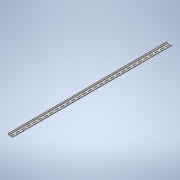
# Autodesk Inventor part: TrilhoDIN_Furado_1m
Saved by Autodesk Inventor 2021 (Build 250183000, 183)
## iProperties
Created: 2022-06-08
Part Number: TrilhoDIN_Furado_1m
Material: Generic
Document SubType Name: Sheet Metal
Designer: danie
Density: 1 g/cm^3
Sheet Metal Rule: Default_mm
Appearance: Default
Author: danie
Autodesk Inventor part; units mm, degrees
(part 1 of 2)
ref_plane "YZ Plane" through (0, 0, 0) normal (1, 0, 0) x (0, 1, 0)
ref_plane "XZ Plane" through (0, 0, 0) normal (0, 1, 0) x (-1, 0, 0)
ref_plane "XY Plane" through (0, 0, 0) normal (0, 0, 1) x (1, 0, 0)
sketch "Sketch1" plane through (0, 0, 0) normal (0, 1, 0) x (-1, 0, 0)
  line L0 (-13.5, 500) -> (13.5, 500)
  line L1 (13.5, 500) -> (13.5, -500)
  line L2 (13.5, -500) -> (-13.5, -500)
  line L3 (-13.5, -500) -> (-13.5, 500)
  line L4 (-13.5, 500) -> (13.5, -500) construction
  line L5 (13.5, 500) -> (-13.5, -500) construction
  point P0 (0, 0)
  dimension "d0" = 27
  dimension "d1" = 1000
  measures "d0" distance of L1.end L2.end
  measures "d1" distance of L0.end L1.end
extrude "Plate1" add sketch "Sketch1" along normal blind 1.5
sketch "Sketch2" plane through (12, 0, -500) normal (1, 0, 0) x (0, 1, 0)
  line L0 (0, 1000) -> (0, 0)
  line L1 (0, 0) -> (7.3, 0)
  line L2 (7.3, 0) -> (7.3, 1000)
  line L3 (7.3, 1000) -> (0, 1000)
  constraints: 6 end point, 1 horizontal, 1 perpendicular, 1 vertical
edge flange "Flange1" height 7.3 angle 90 thickness 1.5 bend radius 1.5 thickness toward (1, 0, 0) relief tear relief width 1.5 relief depth 0.75 corner gap 1.5 corner form 0 edges at (13.5, 1.5, 0) (-13.5, 1.5, 0) wall of the first edge with corners at (12, 0, 500) (12, 0, -500) (12, 7.3, -500) (12, 7.3, 500)
bend "Bend1"
corner "Corner1"
sketch "Sketch3" plane through (12, 5.8, 500) normal (0, 1, 0) x (-1, 0, 0)
  line L0 (0, -1000) -> (0, 0)
  line L1 (0, 0) -> (-5.5, 0)
  line L2 (-5.5, 0) -> (-5.5, -1000)
  line L3 (-5.5, -1000) -> (0, -1000)
  constraints: 6 end point, 1 horizontal, 1 perpendicular, 1 vertical
edge flange "Flange2" height 5.5 angle 90 thickness 1.5 bend radius 1.5 thickness toward (0, 1, 0) relief tear relief width 1.5 relief depth 0.75 corner gap 1.5 corner form 0 edges at (13.5, 7.3, 0) (-13.5, 7.3, 0) wall of the first edge with corners at (12, 5.8, -500) (12, 5.8, 500) (17.5, 5.8, 500) (17.5, 5.8, -500)
bend "Bend2"
corner "Corner2"
sketch "Sketch4" plane through (0, 1.5, 0) normal (0, 1, 0) x (1, 0, 0)
  line L0 (0, -10.25) -> (0, 10.25) construction
  line L1 (2.25, -10.25) -> (2.25, 10.25)
  line L2 (-2.25, 10.25) -> (-2.25, -10.25)
  arc A0 (-2.25, -10.25) -> (2.25, -10.25) centre (0, -10.25) ccw
  arc A1 (2.25, 10.25) -> (-2.25, 10.25) centre (0, 10.25) ccw
  line L3 (0, 24.75) -> (0, 45.25) construction
  line L4 (2.25, 24.75) -> (2.25, 45.25)
  line L5 (-2.25, 45.25) -> (-2.25, 24.75)
  arc A2 (-2.25, 24.75) -> (2.25, 24.75) centre (0, 24.75) ccw
  arc A3 (2.25, 45.25) -> (-2.25, 45.25) centre (0, 45.25) ccw
  line L6 (0, 59.75) -> (0, 80.25) construction
  line L7 (2.25, 59.75) -> (2.25, 80.25)
  line L8 (-2.25, 80.25) -> (-2.25, 59.75)
  arc A4 (-2.25, 59.75) -> (2.25, 59.75) centre (0, 59.75) ccw
  arc A5 (2.25, 80.25) -> (-2.25, 80.25) centre (0, 80.25) ccw
  line L9 (0, 94.75) -> (0, 115.25) construction
  line L10 (2.25, 94.75) -> (2.25, 115.25)
  line L11 (-2.25, 115.25) -> (-2.25, 94.75)
  arc A6 (-2.25, 94.75) -> (2.25, 94.75) centre (0, 94.75) ccw
  arc A7 (2.25, 115.25) -> (-2.25, 115.25) centre (0, 115.25) ccw
  line L12 (0, 129.75) -> (0, 150.25) construction
  line L13 (2.25, 129.75) -> (2.25, 150.25)
  line L14 (-2.25, 150.25) -> (-2.25, 129.75)
  arc A8 (-2.25, 129.75) -> (2.25, 129.75) centre (0, 129.75) ccw
  arc A9 (2.25, 150.25) -> (-2.25, 150.25) centre (0, 150.25) ccw
  line L15 (0, 164.75) -> (0, 185.25) construction
  line L16 (2.25, 164.75) -> (2.25, 185.25)
  line L17 (-2.25, 185.25) -> (-2.25, 164.75)
  arc A10 (-2.25, 164.75) -> (2.25, 164.75) centre (0, 164.75) ccw
  arc A11 (2.25, 185.25) -> (-2.25, 185.25) centre (0, 185.25) ccw
  line L18 (0, 199.75) -> (0, 220.25) construction
  line L19 (2.25, 199.75) -> (2.25, 220.25)
  line L20 (-2.25, 220.25) -> (-2.25, 199.75)
  arc A12 (-2.25, 199.75) -> (2.25, 199.75) centre (0, 199.75) ccw
  arc A13 (2.25, 220.25) -> (-2.25, 220.25) centre (0, 220.25) ccw
  line L21 (0, 234.75) -> (0, 255.25) construction
  line L22 (2.25, 234.75) -> (2.25, 255.25)
  line L23 (-2.25, 255.25) -> (-2.25, 234.75)
  arc A14 (-2.25, 234.75) -> (2.25, 234.75) centre (0, 234.75) ccw
  arc A15 (2.25, 255.25) -> (-2.25, 255.25) centre (0, 255.25) ccw
  line L24 (0, 269.75) -> (0, 290.25) construction
  line L25 (2.25, 269.75) -> (2.25, 290.25)
  line L26 (-2.25, 290.25) -> (-2.25, 269.75)
  arc A16 (-2.25, 269.75) -> (2.25, 269.75) centre (0, 269.75) ccw
  arc A17 (2.25, 290.25) -> (-2.25, 290.25) centre (0, 290.25) ccw
  line L27 (0, 304.75) -> (0, 325.25) construction
  line L28 (2.25, 304.75) -> (2.25, 325.25)
  line L29 (-2.25, 325.25) -> (-2.25, 304.75)
  arc A18 (-2.25, 304.75) -> (2.25, 304.75) centre (0, 304.75) ccw
  arc A19 (2.25, 325.25) -> (-2.25, 325.25) centre (0, 325.25) ccw
  line L30 (0, 339.75) -> (0, 360.25) construction
  line L31 (2.25, 339.75) -> (2.25, 360.25)
  line L32 (-2.25, 360.25) -> (-2.25, 339.75)
  arc A20 (-2.25, 339.75) -> (2.25, 339.75) centre (0, 339.75) ccw
  arc A21 (2.25, 360.25) -> (-2.25, 360.25) centre (0, 360.25) ccw
  line L33 (0, 374.75) -> (0, 395.25) construction
  line L34 (2.25, 374.75) -> (2.25, 395.25)
  line L35 (-2.25, 395.25) -> (-2.25, 374.75)
  arc A22 (-2.25, 374.75) -> (2.25, 374.75) centre (0, 374.75) ccw
  arc A23 (2.25, 395.25) -> (-2.25, 395.25) centre (0, 395.25) ccw
  line L36 (0, 409.75) -> (0, 430.25) construction
  line L37 (2.25, 409.75) -> (2.25, 430.25)
  line L38 (-2.25, 430.25) -> (-2.25, 409.75)
  arc A24 (-2.25, 409.75) -> (2.25, 409.75) centre (0, 409.75) ccw
  arc A25 (2.25, 430.25) -> (-2.25, 430.25) centre (0, 430.25) ccw
  line L39 (0, 444.75) -> (0, 465.25) construction
  line L40 (2.25, 444.75) -> (2.25, 465.25)
  line L41 (-2.25, 465.25) -> (-2.25, 444.75)
  arc A26 (-2.25, 444.75) -> (2.25, 444.75) centre (0, 444.75) ccw
  arc A27 (2.25, 465.25) -> (-2.25, 465.25) centre (0, 465.25) ccw
  line L42 (0, -45.25) -> (0, -24.75) construction
  line L43 (2.25, -45.25) -> (2.25, -24.75)
  line L44 (-2.25, -24.75) -> (-2.25, -45.25)
  arc A28 (-2.25, -45.25) -> (2.25, -45.25) centre (0, -45.25) ccw
  arc A29 (2.25, -24.75) -> (-2.25, -24.75) centre (0, -24.75) ccw
  line L45 (0, -10.25) -> (0, 10.25) construction
  line L46 (2.25, -10.25) -> (2.25, 10.25)
  line L47 (-2.25, 10.25) -> (-2.25, -10.25)
  arc A30 (-2.25, -10.25) -> (2.25, -10.25) centre (0, -10.25) ccw
  arc A31 (2.25, 10.25) -> (-2.25, 10.25) centre (0, 10.25) ccw
  line L48 (0, 24.75) -> (0, 45.25) construction
  line L49 (2.25, 24.75) -> (2.25, 45.25)
  line L50 (-2.25, 45.25) -> (-2.25, 24.75)
  arc A32 (-2.25, 24.75) -> (2.25, 24.75) centre (0, 24.75) ccw
  arc A33 (2.25, 45.25) -> (-2.25, 45.25) centre (0, 45.25) ccw
  line L51 (0, 59.75) -> (0, 80.25) construction
  line L52 (2.25, 59.75) -> (2.25, 80.25)
  line L53 (-2.25, 80.25) -> (-2.25, 59.75)
  arc A34 (-2.25, 59.75) -> (2.25, 59.75) centre (0, 59.75) ccw
  arc A35 (2.25, 80.25) -> (-2.25, 80.25) centre (0, 80.25) ccw
  line L54 (0, 94.75) -> (0, 115.25) construction
  line L55 (2.25, 94.75) -> (2.25, 115.25)
  line L56 (-2.25, 115.25) -> (-2.25, 94.75)
  arc A36 (-2.25, 94.75) -> (2.25, 94.75) centre (0, 94.75) ccw
  arc A37 (2.25, 115.25) -> (-2.25, 115.25) centre (0, 115.25) ccw
  line L57 (0, 129.75) -> (0, 150.25) construction
  line L58 (2.25, 129.75) -> (2.25, 150.25)
  line L59 (-2.25, 150.25) -> (-2.25, 129.75)
  arc A38 (-2.25, 129.75) -> (2.25, 129.75) centre (0, 129.75) ccw
  arc A39 (2.25, 150.25) -> (-2.25, 150.25) centre (0, 150.25) ccw
  line L60 (0, 164.75) -> (0, 185.25) construction
  line L61 (2.25, 164.75) -> (2.25, 185.25)
  line L62 (-2.25, 185.25) -> (-2.25, 164.75)
  arc A40 (-2.25, 164.75) -> (2.25, 164.75) centre (0, 164.75) ccw
  arc A41 (2.25, 185.25) -> (-2.25, 185.25) centre (0, 185.25) ccw
  line L63 (0, 199.75) -> (0, 220.25) construction
  line L64 (2.25, 199.75) -> (2.25, 220.25)
  line L65 (-2.25, 220.25) -> (-2.25, 199.75)
  arc A42 (-2.25, 199.75) -> (2.25, 199.75) centre (0, 199.75) ccw
  arc A43 (2.25, 220.25) -> (-2.25, 220.25) centre (0, 220.25) ccw
  line L66 (0, 234.75) -> (0, 255.25) construction
  line L67 (2.25, 234.75) -> (2.25, 255.25)
  line L68 (-2.25, 255.25) -> (-2.25, 234.75)
  arc A44 (-2.25, 234.75) -> (2.25, 234.75) centre (0, 234.75) ccw
  arc A45 (2.25, 255.25) -> (-2.25, 255.25) centre (0, 255.25) ccw
  line L69 (0, 269.75) -> (0, 290.25) construction
  line L70 (2.25, 269.75) -> (2.25, 290.25)
  line L71 (-2.25, 290.25) -> (-2.25, 269.75)
  arc A46 (-2.25, 269.75) -> (2.25, 269.75) centre (0, 269.75) ccw
  arc A47 (2.25, 290.25) -> (-2.25, 290.25) centre (0, 290.25) ccw
  line L72 (0, 304.75) -> (0, 325.25) construction
  line L73 (2.25, 304.75) -> (2.25, 325.25)
  line L74 (-2.25, 325.25) -> (-2.25, 304.75)
  arc A48 (-2.25, 304.75) -> (2.25, 304.75) centre (0, 304.75) ccw
  arc A49 (2.25, 325.25) -> (-2.25, 325.25) centre (0, 325.25) ccw
  line L75 (0, 339.75) -> (0, 360.25) construction
  line L76 (2.25, 339.75) -> (2.25, 360.25)
  line L77 (-2.25, 360.25) -> (-2.25, 339.75)
  arc A50 (-2.25, 339.75) -> (2.25, 339.75) centre (0, 339.75) ccw
  arc A51 (2.25, 360.25) -> (-2.25, 360.25) centre (0, 360.25) ccw
  line L78 (0, 374.75) -> (0, 395.25) construction
  line L79 (2.25, 374.75) -> (2.25, 395.25)
  line L80 (-2.25, 395.25) -> (-2.25, 374.75)
  arc A52 (-2.25, 374.75) -> (2.25, 374.75) centre (0, 374.75) ccw
  arc A53 (2.25, 395.25) -> (-2.25, 395.25) centre (0, 395.25) ccw
  line L81 (0, 409.75) -> (0, 430.25) construction
  line L82 (2.25, 409.75) -> (2.25, 430.25)
  line L83 (-2.25, 430.25) -> (-2.25, 409.75)
  arc A54 (-2.25, 409.75) -> (2.25, 409.75) centre (0, 409.75) ccw
  arc A55 (2.25, 430.25) -> (-2.25, 430.25) centre (0, 430.25) ccw
  line L84 (0, -80.25) -> (0, -59.75) construction
  line L85 (2.25, -80.25) -> (2.25, -59.75)
  line L86 (-2.25, -59.75) -> (-2.25, -80.25)
  arc A56 (-2.25, -80.25) -> (2.25, -80.25) centre (0, -80.25) ccw
  arc A57 (2.25, -59.75) -> (-2.25, -59.75) centre (0, -59.75) ccw
  line L87 (0, -45.25) -> (0, -24.75) construction
  line L88 (2.25, -45.25) -> (2.25, -24.75)
  line L89 (-2.25, -24.75) -> (-2.25, -45.25)
  arc A58 (-2.25, -45.25) -> (2.25, -45.25) centre (0, -45.25) ccw
  arc A59 (2.25, -24.75) -> (-2.25, -24.75) centre (0, -24.75) ccw
  line L90 (0, -10.25) -> (0, 10.25) construction
  line L91 (2.25, -10.25) -> (2.25, 10.25)
  line L92 (-2.25, 10.25) -> (-2.25, -10.25)
  arc A60 (-2.25, -10.25) -> (2.25, -10.25) centre (0, -10.25) ccw
  arc A61 (2.25, 10.25) -> (-2.25, 10.25) centre (0, 10.25) ccw
  line L93 (0, 24.75) -> (0, 45.25) construction
  line L94 (2.25, 24.75) -> (2.25, 45.25)
  line L95 (-2.25, 45.25) -> (-2.25, 24.75)
  arc A62 (-2.25, 24.75) -> (2.25, 24.75) centre (0, 24.75) ccw
  arc A63 (2.25, 45.25) -> (-2.25, 45.25) centre (0, 45.25) ccw
  line L96 (0, 59.75) -> (0, 80.25) construction
  line L97 (2.25, 59.75) -> (2.25, 80.25)
  line L98 (-2.25, 80.25) -> (-2.25, 59.75)
  arc A64 (-2.25, 59.75) -> (2.25, 59.75) centre (0, 59.75) ccw
  arc A65 (2.25, 80.25) -> (-2.25, 80.25) centre (0, 80.25) ccw
  line L99 (0, 94.75) -> (0, 115.25) construction
  line L100 (2.25, 94.75) -> (2.25, 115.25)
  line L101 (-2.25, 115.25) -> (-2.25, 94.75)
  arc A66 (-2.25, 94.75) -> (2.25, 94.75) centre (0, 94.75) ccw
  arc A67 (2.25, 115.25) -> (-2.25, 115.25) centre (0, 115.25) ccw
  line L102 (0, 129.75) -> (0, 150.25) construction
  line L103 (2.25, 129.75) -> (2.25, 150.25)
  line L104 (-2.25, 150.25) -> (-2.25, 129.75)
  arc A68 (-2.25, 129.75) -> (2.25, 129.75) centre (0, 129.75) ccw
  arc A69 (2.25, 150.25) -> (-2.25, 150.25) centre (0, 150.25) ccw
  line L105 (0, 164.75) -> (0, 185.25) construction
  line L106 (2.25, 164.75) -> (2.25, 185.25)
  line L107 (-2.25, 185.25) -> (-2.25, 164.75)
  arc A70 (-2.25, 164.75) -> (2.25, 164.75) centre (0, 164.75) ccw
  arc A71 (2.25, 185.25) -> (-2.25, 185.25) centre (0, 185.25) ccw
  line L108 (0, 199.75) -> (0, 220.25) construction
  line L109 (2.25, 199.75) -> (2.25, 220.25)
  line L110 (-2.25, 220.25) -> (-2.25, 199.75)
  arc A72 (-2.25, 199.75) -> (2.25, 199.75) centre (0, 199.75) ccw
  arc A73 (2.25, 220.25) -> (-2.25, 220.25) centre (0, 220.25) ccw
  line L111 (0, 234.75) -> (0, 255.25) construction
  line L112 (2.25, 234.75) -> (2.25, 255.25)
  line L113 (-2.25, 255.25) -> (-2.25, 234.75)
  arc A74 (-2.25, 234.75) -> (2.25, 234.75) centre (0, 234.75) ccw
  arc A75 (2.25, 255.25) -> (-2.25, 255.25) centre (0, 255.25) ccw
  line L114 (0, 269.75) -> (0, 290.25) construction
  line L115 (2.25, 269.75) -> (2.25, 290.25)
  line L116 (-2.25, 290.25) -> (-2.25, 269.75)
  arc A76 (-2.25, 269.75) -> (2.25, 269.75) centre (0, 269.75) ccw
  arc A77 (2.25, 290.25) -> (-2.25, 290.25) centre (0, 290.25) ccw
  line L117 (0, 304.75) -> (0, 325.25) construction
  line L118 (2.25, 304.75) -> (2.25, 325.25)
  line L119 (-2.25, 325.25) -> (-2.25, 304.75)
  arc A78 (-2.25, 304.75) -> (2.25, 304.75) centre (0, 304.75) ccw
  arc A79 (2.25, 325.25) -> (-2.25, 325.25) centre (0, 325.25) ccw
  line L120 (0, 339.75) -> (0, 360.25) construction
  line L121 (2.25, 339.75) -> (2.25, 360.25)
  line L122 (-2.25, 360.25) -> (-2.25, 339.75)
  arc A80 (-2.25, 339.75) -> (2.25, 339.75) centre (0, 339.75) ccw
  arc A81 (2.25, 360.25) -> (-2.25, 360.25) centre (0, 360.25) ccw
  line L123 (0, 374.75) -> (0, 395.25) construction
  line L124 (2.25, 374.75) -> (2.25, 395.25)
  line L125 (-2.25, 395.25) -> (-2.25, 374.75)
  arc A82 (-2.25, 374.75) -> (2.25, 374.75) centre (0, 374.75) ccw
  arc A83 (2.25, 395.25) -> (-2.25, 395.25) centre (0, 395.25) ccw
  line L126 (0, -115.25) -> (0, -94.75) construction
  line L127 (2.25, -115.25) -> (2.25, -94.75)
  line L128 (-2.25, -94.75) -> (-2.25, -115.25)
  arc A84 (-2.25, -115.25) -> (2.25, -115.25) centre (0, -115.25) ccw
  arc A85 (2.25, -94.75) -> (-2.25, -94.75) centre (0, -94.75) ccw
  line L129 (0, -80.25) -> (0, -59.75) construction
  line L130 (2.25, -80.25) -> (2.25, -59.75)
  line L131 (-2.25, -59.75) -> (-2.25, -80.25)
  arc A86 (-2.25, -80.25) -> (2.25, -80.25) centre (0, -80.25) ccw
  arc A87 (2.25, -59.75) -> (-2.25, -59.75) centre (0, -59.75) ccw
  line L132 (0, -45.25) -> (0, -24.75) construction
  line L133 (2.25, -45.25) -> (2.25, -24.75)
  line L134 (-2.25, -24.75) -> (-2.25, -45.25)
  arc A88 (-2.25, -45.25) -> (2.25, -45.25) centre (0, -45.25) ccw
  arc A89 (2.25, -24.75) -> (-2.25, -24.75) centre (0, -24.75) ccw
  line L135 (0, -10.25) -> (0, 10.25) construction
  line L136 (2.25, -10.25) -> (2.25, 10.25)
  line L137 (-2.25, 10.25) -> (-2.25, -10.25)
  arc A90 (-2.25, -10.25) -> (2.25, -10.25) centre (0, -10.25) ccw
  arc A91 (2.25, 10.25) -> (-2.25, 10.25) centre (0, 10.25) ccw
  line L138 (0, 24.75) -> (0, 45.25) construction
  line L139 (2.25, 24.75) -> (2.25, 45.25)
  line L140 (-2.25, 45.25) -> (-2.25, 24.75)
  arc A92 (-2.25, 24.75) -> (2.25, 24.75) centre (0, 24.75) ccw
  arc A93 (2.25, 45.25) -> (-2.25, 45.25) centre (0, 45.25) ccw
  line L141 (0, 59.75) -> (0, 80.25) construction
  line L142 (2.25, 59.75) -> (2.25, 80.25)
  line L143 (-2.25, 80.25) -> (-2.25, 59.75)
  arc A94 (-2.25, 59.75) -> (2.25, 59.75) centre (0, 59.75) ccw
  arc A95 (2.25, 80.25) -> (-2.25, 80.25) centre (0, 80.25) ccw
  line L144 (0, 94.75) -> (0, 115.25) construction
  line L145 (2.25, 94.75) -> (2.25, 115.25)
  line L146 (-2.25, 115.25) -> (-2.25, 94.75)
  arc A96 (-2.25, 94.75) -> (2.25, 94.75) centre (0, 94.75) ccw
  arc A97 (2.25, 115.25) -> (-2.25, 115.25) centre (0, 115.25) ccw
  line L147 (0, 129.75) -> (0, 150.25) construction
  line L148 (2.25, 129.75) -> (2.25, 150.25)
  line L149 (-2.25, 150.25) -> (-2.25, 129.75)
  arc A98 (-2.25, 129.75) -> (2.25, 129.75) centre (0, 129.75) ccw
  arc A99 (2.25, 150.25) -> (-2.25, 150.25) centre (0, 150.25) ccw
  line L150 (0, 164.75) -> (0, 185.25) construction
  line L151 (2.25, 164.75) -> (2.25, 185.25)
  line L152 (-2.25, 185.25) -> (-2.25, 164.75)
  arc A100 (-2.25, 164.75) -> (2.25, 164.75) centre (0, 164.75) ccw
  arc A101 (2.25, 185.25) -> (-2.25, 185.25) centre (0, 185.25) ccw
  line L153 (0, 199.75) -> (0, 220.25) construction
  line L154 (2.25, 199.75) -> (2.25, 220.25)
  line L155 (-2.25, 220.25) -> (-2.25, 199.75)
  arc A102 (-2.25, 199.75) -> (2.25, 199.75) centre (0, 199.75) ccw
  arc A103 (2.25, 220.25) -> (-2.25, 220.25) centre (0, 220.25) ccw
  line L156 (0, 234.75) -> (0, 255.25) construction
  line L157 (2.25, 234.75) -> (2.25, 255.25)
  line L158 (-2.25, 255.25) -> (-2.25, 234.75)
  arc A104 (-2.25, 234.75) -> (2.25, 234.75) centre (0, 234.75) ccw
  arc A105 (2.25, 255.25) -> (-2.25, 255.25) centre (0, 255.25) ccw
  line L159 (0, 269.75) -> (0, 290.25) construction
  line L160 (2.25, 269.75) -> (2.25, 290.25)
  line L161 (-2.25, 290.25) -> (-2.25, 269.75)
  arc A106 (-2.25, 269.75) -> (2.25, 269.75) centre (0, 269.75) ccw
  arc A107 (2.25, 290.25) -> (-2.25, 290.25) centre (0, 290.25) ccw
  line L162 (0, 304.75) -> (0, 325.25) construction
  line L163 (2.25, 304.75) -> (2.25, 325.25)
  line L164 (-2.25, 325.25) -> (-2.25, 304.75)
  arc A108 (-2.25, 304.75) -> (2.25, 304.75) centre (0, 304.75) ccw
  arc A109 (2.25, 325.25) -> (-2.25, 325.25) centre (0, 325.25) ccw
  line L165 (0, 339.75) -> (0, 360.25) construction
  line L166 (2.25, 339.75) -> (2.25, 360.25)
  line L167 (-2.25, 360.25) -> (-2.25, 339.75)
  arc A110 (-2.25, 339.75) -> (2.25, 339.75) centre (0, 339.75) ccw
  arc A111 (2.25, 360.25) -> (-2.25, 360.25) centre (0, 360.25) ccw
  line L168 (0, -150.25) -> (0, -129.75) construction
  line L169 (2.25, -150.25) -> (2.25, -129.75)
  line L170 (-2.25, -129.75) -> (-2.25, -150.25)
  arc A112 (-2.25, -150.25) -> (2.25, -150.25) centre (0, -150.25) ccw
  arc A113 (2.25, -129.75) -> (-2.25, -129.75) centre (0, -129.75) ccw
  line L171 (0, -115.25) -> (0, -94.75) construction
  line L172 (2.25, -115.25) -> (2.25, -94.75)
  line L173 (-2.25, -94.75) -> (-2.25, -115.25)
  arc A114 (-2.25, -115.25) -> (2.25, -115.25) centre (0, -115.25) ccw
  arc A115 (2.25, -94.75) -> (-2.25, -94.75) centre (0, -94.75) ccw
  line L174 (0, -80.25) -> (0, -59.75) construction
  line L175 (2.25, -80.25) -> (2.25, -59.75)
  line L176 (-2.25, -59.75) -> (-2.25, -80.25)
  arc A116 (-2.25, -80.25) -> (2.25, -80.25) centre (0, -80.25) ccw
  arc A117 (2.25, -59.75) -> (-2.25, -59.75) centre (0, -59.75) ccw
  line L177 (0, -45.25) -> (0, -24.75) construction
  line L178 (2.25, -45.25) -> (2.25, -24.75)
  line L179 (-2.25, -24.75) -> (-2.25, -45.25)
  arc A118 (-2.25, -45.25) -> (2.25, -45.25) centre (0, -45.25) ccw
  arc A119 (2.25, -24.75) -> (-2.25, -24.75) centre (0, -24.75) ccw
  line L180 (0, -10.25) -> (0, 10.25) construction
  line L181 (2.25, -10.25) -> (2.25, 10.25)
  line L182 (-2.25, 10.25) -> (-2.25, -10.25)
  arc A120 (-2.25, -10.25) -> (2.25, -10.25) centre (0, -10.25) ccw
  arc A121 (2.25, 10.25) -> (-2.25, 10.25) centre (0, 10.25) ccw
  line L183 (0, 24.75) -> (0, 45.25) construction
  line L184 (2.25, 24.75) -> (2.25, 45.25)
  line L185 (-2.25, 45.25) -> (-2.25, 24.75)
  arc A122 (-2.25, 24.75) -> (2.25, 24.75) centre (0, 24.75) ccw
  arc A123 (2.25, 45.25) -> (-2.25, 45.25) centre (0, 45.25) ccw
  line L186 (0, 59.75) -> (0, 80.25) construction
  line L187 (2.25, 59.75) -> (2.25, 80.25)
  line L188 (-2.25, 80.25) -> (-2.25, 59.75)
  arc A124 (-2.25, 59.75) -> (2.25, 59.75) centre (0, 59.75) ccw
  arc A125 (2.25, 80.25) -> (-2.25, 80.25) centre (0, 80.25) ccw
  line L189 (0, 94.75) -> (0, 115.25) construction
  line L190 (2.25, 94.75) -> (2.25, 115.25)
  line L191 (-2.25, 115.25) -> (-2.25, 94.75)
  arc A126 (-2.25, 94.75) -> (2.25, 94.75) centre (0, 94.75) ccw
  arc A127 (2.25, 115.25) -> (-2.25, 115.25) centre (0, 115.25) ccw
  line L192 (0, 129.75) -> (0, 150.25) construction
  line L193 (2.25, 129.75) -> (2.25, 150.25)
  line L194 (-2.25, 150.25) -> (-2.25, 129.75)
  arc A128 (-2.25, 129.75) -> (2.25, 129.75) centre (0, 129.75) ccw
  arc A129 (2.25, 150.25) -> (-2.25, 150.25) centre (0, 150.25) ccw
  line L195 (0, 164.75) -> (0, 185.25) construction
  line L196 (2.25, 164.75) -> (2.25, 185.25)
  line L197 (-2.25, 185.25) -> (-2.25, 164.75)
  arc A130 (-2.25, 164.75) -> (2.25, 164.75) centre (0, 164.75) ccw
  arc A131 (2.25, 185.25) -> (-2.25, 185.25) centre (0, 185.25) ccw
  line L198 (0, 199.75) -> (0, 220.25) construction
  line L199 (2.25, 199.75) -> (2.25, 220.25)
  line L200 (-2.25, 220.25) -> (-2.25, 199.75)
  arc A132 (-2.25, 199.75) -> (2.25, 199.75) centre (0, 199.75) ccw
  arc A133 (2.25, 220.25) -> (-2.25, 220.25) centre (0, 220.25) ccw
  line L201 (0, 234.75) -> (0, 255.25) construction
  line L202 (2.25, 234.75) -> (2.25, 255.25)
  line L203 (-2.25, 255.25) -> (-2.25, 234.75)
  arc A134 (-2.25, 234.75) -> (2.25, 234.75) centre (0, 234.75) ccw
  arc A135 (2.25, 255.25) -> (-2.25, 255.25) centre (0, 255.25) ccw
  line L204 (0, 269.75) -> (0, 290.25) construction
  line L205 (2.25, 269.75) -> (2.25, 290.25)
  line L206 (-2.25, 290.25) -> (-2.25, 269.75)
  arc A136 (-2.25, 269.75) -> (2.25, 269.75) centre (0, 269.75) ccw
  arc A137 (2.25, 290.25) -> (-2.25, 290.25) centre (0, 290.25) ccw
  line L207 (0, 304.75) -> (0, 325.25) construction
  line L208 (2.25, 304.75) -> (2.25, 325.25)
  line L209 (-2.25, 325.25) -> (-2.25, 304.75)
  arc A138 (-2.25, 304.75) -> (2.25, 304.75) centre (0, 304.75) ccw
  arc A139 (2.25, 325.25) -> (-2.25, 325.25) centre (0, 325.25) ccw
  line L210 (0, -185.25) -> (0, -164.75) construction
  line L211 (2.25, -185.25) -> (2.25, -164.75)
  line L212 (-2.25, -164.75) -> (-2.25, -185.25)
  arc A140 (-2.25, -185.25) -> (2.25, -185.25) centre (0, -185.25) ccw
  arc A141 (2.25, -164.75) -> (-2.25, -164.75) centre (0, -164.75) ccw
  line L213 (0, -150.25) -> (0, -129.75) construction
  line L214 (2.25, -150.25) -> (2.25, -129.75)
  line L215 (-2.25, -129.75) -> (-2.25, -150.25)
  arc A142 (-2.25, -150.25) -> (2.25, -150.25) centre (0, -150.25) ccw
  arc A143 (2.25, -129.75) -> (-2.25, -129.75) centre (0, -129.75) ccw
  line L216 (0, -115.25) -> (0, -94.75) construction
  line L217 (2.25, -115.25) -> (2.25, -94.75)
  line L218 (-2.25, -94.75) -> (-2.25, -115.25)
  arc A144 (-2.25, -115.25) -> (2.25, -115.25) centre (0, -115.25) ccw
  arc A145 (2.25, -94.75) -> (-2.25, -94.75) centre (0, -94.75) ccw
  line L219 (0, -80.25) -> (0, -59.75) construction
  line L220 (2.25, -80.25) -> (2.25, -59.75)
  line L221 (-2.25, -59.75) -> (-2.25, -80.25)
  arc A146 (-2.25, -80.25) -> (2.25, -80.25) centre (0, -80.25) ccw
  arc A147 (2.25, -59.75) -> (-2.25, -59.75) centre (0, -59.75) ccw
  line L222 (0, -45.25) -> (0, -24.75) construction
  line L223 (2.25, -45.25) -> (2.25, -24.75)
  line L224 (-2.25, -24.75) -> (-2.25, -45.25)
  arc A148 (-2.25, -45.25) -> (2.25, -45.25) centre (0, -45.25) ccw
  arc A149 (2.25, -24.75) -> (-2.25, -24.75) centre (0, -24.75) ccw
  line L225 (0, -10.25) -> (0, 10.25) construction
  line L226 (2.25, -10.25) -> (2.25, 10.25)
  line L227 (-2.25, 10.25) -> (-2.25, -10.25)
  arc A150 (-2.25, -10.25) -> (2.25, -10.25) centre (0, -10.25) ccw
  arc A151 (2.25, 10.25) -> (-2.25, 10.25) centre (0, 10.25) ccw
  line L228 (0, 24.75) -> (0, 45.25) construction
  line L229 (2.25, 24.75) -> (2.25, 45.25)
  line L230 (-2.25, 45.25) -> (-2.25, 24.75)
  arc A152 (-2.25, 24.75) -> (2.25, 24.75) centre (0, 24.75) ccw
  arc A153 (2.25, 45.25) -> (-2.25, 45.25) centre (0, 45.25) ccw
  line L231 (0, 59.75) -> (0, 80.25) construction
  line L232 (2.25, 59.75) -> (2.25, 80.25)
  line L233 (-2.25, 80.25) -> (-2.25, 59.75)
  arc A154 (-2.25, 59.75) -> (2.25, 59.75) centre (0, 59.75) ccw
  arc A155 (2.25, 80.25) -> (-2.25, 80.25) centre (0, 80.25) ccw
  line L234 (0, 94.75) -> (0, 115.25) construction
  line L235 (2.25, 94.75) -> (2.25, 115.25)
  line L236 (-2.25, 115.25) -> (-2.25, 94.75)
  arc A156 (-2.25, 94.75) -> (2.25, 94.75) centre (0, 94.75) ccw
  arc A157 (2.25, 115.25) -> (-2.25, 115.25) centre (0, 115.25) ccw
  line L237 (0, 129.75) -> (0, 150.25) construction
  line L238 (2.25, 129.75) -> (2.25, 150.25)
  line L239 (-2.25, 150.25) -> (-2.25, 129.75)
  arc A158 (-2.25, 129.75) -> (2.25, 129.75) centre (0, 129.75) ccw
  arc A159 (2.25, 150.25) -> (-2.25, 150.25) centre (0, 150.25) ccw
  line L240 (0, 164.75) -> (0, 185.25) construction
  line L241 (2.25, 164.75) -> (2.25, 185.25)
  line L242 (-2.25, 185.25) -> (-2.25, 164.75)
  arc A160 (-2.25, 164.75) -> (2.25, 164.75) centre (0, 164.75) ccw
  arc A161 (2.25, 185.25) -> (-2.25, 185.25) centre (0, 185.25) ccw
  line L243 (0, 199.75) -> (0, 220.25) construction
  line L244 (2.25, 199.75) -> (2.25, 220.25)
  line L245 (-2.25, 220.25) -> (-2.25, 199.75)
  arc A162 (-2.25, 199.75) -> (2.25, 199.75) centre (0, 199.75) ccw
  arc A163 (2.25, 220.25) -> (-2.25, 220.25) centre (0, 220.25) ccw
  line L246 (0, 234.75) -> (0, 255.25) construction
  line L247 (2.25, 234.75) -> (2.25, 255.25)
  line L248 (-2.25, 255.25) -> (-2.25, 234.75)
  arc A164 (-2.25, 234.75) -> (2.25, 234.75) centre (0, 234.75) ccw
  arc A165 (2.25, 255.25) -> (-2.25, 255.25) centre (0, 255.25) ccw
  line L249 (0, 269.75) -> (0, 290.25) construction
  line L250 (2.25, 269.75) -> (2.25, 290.25)
  line L251 (-2.25, 290.25) -> (-2.25, 269.75)
  arc A166 (-2.25, 269.75) -> (2.25, 269.75) centre (0, 269.75) ccw
  arc A167 (2.25, 290.25) -> (-2.25, 290.25) centre (0, 290.25) ccw
  line L252 (0, -220.25) -> (0, -199.75) construction
  line L253 (2.25, -220.25) -> (2.25, -199.75)
  line L254 (-2.25, -199.75) -> (-2.25, -220.25)
  arc A168 (-2.25, -220.25) -> (2.25, -220.25) centre (0, -220.25) ccw
  arc A169 (2.25, -199.75) -> (-2.25, -199.75) centre (0, -199.75) ccw
  line L255 (0, -185.25) -> (0, -164.75) construction
  line L256 (2.25, -185.25) -> (2.25, -164.75)
  line L257 (-2.25, -164.75) -> (-2.25, -185.25)
  arc A170 (-2.25, -185.25) -> (2.25, -185.25) centre (0, -185.25) ccw
  arc A171 (2.25, -164.75) -> (-2.25, -164.75) centre (0, -164.75) ccw
  line L258 (0, -150.25) -> (0, -129.75) construction
  line L259 (2.25, -150.25) -> (2.25, -129.75)
  line L260 (-2.25, -129.75) -> (-2.25, -150.25)
  arc A172 (-2.25, -150.25) -> (2.25, -150.25) centre (0, -150.25) ccw
  arc A173 (2.25, -129.75) -> (-2.25, -129.75) centre (0, -129.75) ccw
  line L261 (0, -115.25) -> (0, -94.75) construction
  line L262 (2.25, -115.25) -> (2.25, -94.75)
  line L263 (-2.25, -94.75) -> (-2.25, -115.25)
  arc A174 (-2.25, -115.25) -> (2.25, -115.25) centre (0, -115.25) ccw
  arc A175 (2.25, -94.75) -> (-2.25, -94.75) centre (0, -94.75) ccw
  line L264 (0, -80.25) -> (0, -59.75) construction
  line L265 (2.25, -80.25) -> (2.25, -59.75)
  line L266 (-2.25, -59.75) -> (-2.25, -80.25)
  arc A176 (-2.25, -80.25) -> (2.25, -80.25) centre (0, -80.25) ccw
  arc A177 (2.25, -59.75) -> (-2.25, -59.75) centre (0, -59.75) ccw
  line L267 (0, -45.25) -> (0, -24.75) construction
  line L268 (2.25, -45.25) -> (2.25, -24.75)
  line L269 (-2.25, -24.75) -> (-2.25, -45.25)
  arc A178 (-2.25, -45.25) -> (2.25, -45.25) centre (0, -45.25) ccw
  arc A179 (2.25, -24.75) -> (-2.25, -24.75) centre (0, -24.75) ccw
  line L270 (0, -10.25) -> (0, 10.25) construction
  line L271 (2.25, -10.25) -> (2.25, 10.25)
  line L272 (-2.25, 10.25) -> (-2.25, -10.25)
  arc A180 (-2.25, -10.25) -> (2.25, -10.25) centre (0, -10.25) ccw
  arc A181 (2.25, 10.25) -> (-2.25, 10.25) centre (0, 10.25) ccw
  line L273 (0, 24.75) -> (0, 45.25) construction
  line L274 (2.25, 24.75) -> (2.25, 45.25)
  line L275 (-2.25, 45.25) -> (-2.25, 24.75)
  arc A182 (-2.25, 24.75) -> (2.25, 24.75) centre (0, 24.75) ccw
  arc A183 (2.25, 45.25) -> (-2.25, 45.25) centre (0, 45.25) ccw
  line L276 (0, 59.75) -> (0, 80.25) construction
  line L277 (2.25, 59.75) -> (2.25, 80.25)
  line L278 (-2.25, 80.25) -> (-2.25, 59.75)
  arc A184 (-2.25, 59.75) -> (2.25, 59.75) centre (0, 59.75) ccw
  arc A185 (2.25, 80.25) -> (-2.25, 80.25) centre (0, 80.25) ccw
  line L279 (0, 94.75) -> (0, 115.25) construction
  line L280 (2.25, 94.75) -> (2.25, 115.25)
  line L281 (-2.25, 115.25) -> (-2.25, 94.75)
  arc A186 (-2.25, 94.75) -> (2.25, 94.75) centre (0, 94.75) ccw
  arc A187 (2.25, 115.25) -> (-2.25, 115.25) centre (0, 115.25) ccw
  line L282 (0, 129.75) -> (0, 150.25) construction
  line L283 (2.25, 129.75) -> (2.25, 150.25)
  line L284 (-2.25, 150.25) -> (-2.25, 129.75)
  arc A188 (-2.25, 129.75) -> (2.25, 129.75) centre (0, 129.75) ccw
  arc A189 (2.25, 150.25) -> (-2.25, 150.25) centre (0, 150.25) ccw
  line L285 (0, 164.75) -> (0, 185.25) construction
  line L286 (2.25, 164.75) -> (2.25, 185.25)
  line L287 (-2.25, 185.25) -> (-2.25, 164.75)
  arc A190 (-2.25, 164.75) -> (2.25, 164.75) centre (0, 164.75) ccw
  arc A191 (2.25, 185.25) -> (-2.25, 185.25) centre (0, 185.25) ccw
  line L288 (0, 199.75) -> (0, 220.25) construction
  line L289 (2.25, 199.75) -> (2.25, 220.25)
  line L290 (-2.25, 220.25) -> (-2.25, 199.75)
  arc A192 (-2.25, 199.75) -> (2.25, 199.75) centre (0, 199.75) ccw
  arc A193 (2.25, 220.25) -> (-2.25, 220.25) centre (0, 220.25) ccw
  line L291 (0, 234.75) -> (0, 255.25) construction
  line L292 (2.25, 234.75) -> (2.25, 255.25)
  line L293 (-2.25, 255.25) -> (-2.25, 234.75)
  arc A194 (-2.25, 234.75) -> (2.25, 234.75) centre (0, 234.75) ccw
  arc A195 (2.25, 255.25) -> (-2.25, 255.25) centre (0, 255.25) ccw
  line L294 (0, -255.25) -> (0, -234.75) construction
  line L295 (2.25, -255.25) -> (2.25, -234.75)
  line L296 (-2.25, -234.75) -> (-2.25, -255.25)
  arc A196 (-2.25, -255.25) -> (2.25, -255.25) centre (0, -255.25) ccw
  arc A197 (2.25, -234.75) -> (-2.25, -234.75) centre (0, -234.75) ccw
  line L297 (0, -220.25) -> (0, -199.75) construction
  line L298 (2.25, -220.25) -> (2.25, -199.75)
  line L299 (-2.25, -199.75) -> (-2.25, -220.25)
  arc A198 (-2.25, -220.25) -> (2.25, -220.25) centre (0, -220.25) ccw
  arc A199 (2.25, -199.75) -> (-2.25, -199.75) centre (0, -199.75) ccw
  line L300 (0, -185.25) -> (0, -164.75) construction
  line L301 (2.25, -185.25) -> (2.25, -164.75)
  line L302 (-2.25, -164.75) -> (-2.25, -185.25)
  arc A200 (-2.25, -185.25) -> (2.25, -185.25) centre (0, -185.25) ccw
  arc A201 (2.25, -164.75) -> (-2.25, -164.75) centre (0, -164.75) ccw
  line L303 (0, -150.25) -> (0, -129.75) construction
  line L304 (2.25, -150.25) -> (2.25, -129.75)
  line L305 (-2.25, -129.75) -> (-2.25, -150.25)
  arc A202 (-2.25, -150.25) -> (2.25, -150.25) centre (0, -150.25) ccw
  arc A203 (2.25, -129.75) -> (-2.25, -129.75) centre (0, -129.75) ccw
  line L306 (0, -115.25) -> (0, -94.75) construction
  line L307 (2.25, -115.25) -> (2.25, -94.75)
  line L308 (-2.25, -94.75) -> (-2.25, -115.25)
  arc A204 (-2.25, -115.25) -> (2.25, -115.25) centre (0, -115.25) ccw
  arc A205 (2.25, -94.75) -> (-2.25, -94.75) centre (0, -94.75) ccw
  line L309 (0, -80.25) -> (0, -59.75) construction
  line L310 (2.25, -80.25) -> (2.25, -59.75)
  line L311 (-2.25, -59.75) -> (-2.25, -80.25)
  arc A206 (-2.25, -80.25) -> (2.25, -80.25) centre (0, -80.25) ccw
  arc A207 (2.25, -59.75) -> (-2.25, -59.75) centre (0, -59.75) ccw
  line L312 (0, -45.25) -> (0, -24.75) construction
  line L313 (2.25, -45.25) -> (2.25, -24.75)
  line L314 (-2.25, -24.75) -> (-2.25, -45.25)
  arc A208 (-2.25, -45.25) -> (2.25, -45.25) centre (0, -45.25) ccw
  arc A209 (2.25, -24.75) -> (-2.25, -24.75) centre (0, -24.75) ccw
  line L315 (0, -10.25) -> (0, 10.25) construction
  line L316 (2.25, -10.25) -> (2.25, 10.25)
  line L317 (-2.25, 10.25) -> (-2.25, -10.25)
  arc A210 (-2.25, -10.25) -> (2.25, -10.25) centre (0, -10.25) ccw
  arc A211 (2.25, 10.25) -> (-2.25, 10.25) centre (0, 10.25) ccw
  line L318 (0, 24.75) -> (0, 45.25) construction
  line L319 (2.25, 24.75) -> (2.25, 45.25)
  line L320 (-2.25, 45.25) -> (-2.25, 24.75)
  arc A212 (-2.25, 24.75) -> (2.25, 24.75) centre (0, 24.75) ccw
  arc A213 (2.25, 45.25) -> (-2.25, 45.25) centre (0, 45.25) ccw
  line L321 (0, 59.75) -> (0, 80.25) construction
  line L322 (2.25, 59.75) -> (2.25, 80.25)
  line L323 (-2.25, 80.25) -> (-2.25, 59.75)
  arc A214 (-2.25, 59.75) -> (2.25, 59.75) centre (0, 59.75) ccw
  arc A215 (2.25, 80.25) -> (-2.25, 80.25) centre (0, 80.25) ccw
  line L324 (0, 94.75) -> (0, 115.25) construction
  line L325 (2.25, 94.75) -> (2.25, 115.25)
  line L326 (-2.25, 115.25) -> (-2.25, 94.75)
  arc A216 (-2.25, 94.75) -> (2.25, 94.75) centre (0, 94.75) ccw
  arc A217 (2.25, 115.25) -> (-2.25, 115.25) centre (0, 115.25) ccw
  line L327 (0, 129.75) -> (0, 150.25) construction
  line L328 (2.25, 129.75) -> (2.25, 150.25)
  line L329 (-2.25, 150.25) -> (-2.25, 129.75)
  arc A218 (-2.25, 129.75) -> (2.25, 129.75) centre (0, 129.75) ccw
  arc A219 (2.25, 150.25) -> (-2.25, 150.25) centre (0, 150.25) ccw
  line L330 (0, 164.75) -> (0, 185.25) construction
  line L331 (2.25, 164.75) -> (2.25, 185.25)
  line L332 (-2.25, 185.25) -> (-2.25, 164.75)
  arc A220 (-2.25, 164.75) -> (2.25, 164.75) centre (0, 164.75) ccw
  arc A221 (2.25, 185.25) -> (-2.25, 185.25) centre (0, 185.25) ccw
  line L333 (0, 199.75) -> (0, 220.25) construction
  line L334 (2.25, 199.75) -> (2.25, 220.25)
  line L335 (-2.25, 220.25) -> (-2.25, 199.75)
  arc A222 (-2.25, 199.75) -> (2.25, 199.75) centre (0, 199.75) ccw
  arc A223 (2.25, 220.25) -> (-2.25, 220.25) centre (0, 220.25) ccw
  line L336 (0, -290.25) -> (0, -269.75) construction
  line L337 (2.25, -290.25) -> (2.25, -269.75)
  line L338 (-2.25, -269.75) -> (-2.25, -290.25)
  arc A224 (-2.25, -290.25) -> (2.25, -290.25) centre (0, -290.25) ccw
  arc A225 (2.25, -269.75) -> (-2.25, -269.75) centre (0, -269.75) ccw
  line L339 (0, -255.25) -> (0, -234.75) construction
  line L340 (2.25, -255.25) -> (2.25, -234.75)
  line L341 (-2.25, -234.75) -> (-2.25, -255.25)
  arc A226 (-2.25, -255.25) -> (2.25, -255.25) centre (0, -255.25) ccw
  arc A227 (2.25, -234.75) -> (-2.25, -234.75) centre (0, -234.75) ccw
  line L342 (0, -220.25) -> (0, -199.75) construction
  line L343 (2.25, -220.25) -> (2.25, -199.75)
  line L344 (-2.25, -199.75) -> (-2.25, -220.25)
  arc A228 (-2.25, -220.25) -> (2.25, -220.25) centre (0, -220.25) ccw
  arc A229 (2.25, -199.75) -> (-2.25, -199.75) centre (0, -199.75) ccw
  line L345 (0, -185.25) -> (0, -164.75) construction
  line L346 (2.25, -185.25) -> (2.25, -164.75)
  line L347 (-2.25, -164.75) -> (-2.25, -185.25)
  arc A230 (-2.25, -185.25) -> (2.25, -185.25) centre (0, -185.25) ccw
  arc A231 (2.25, -164.75) -> (-2.25, -164.75) centre (0, -164.75) ccw
  line L348 (0, -150.25) -> (0, -129.75) construction
  line L349 (2.25, -150.25) -> (2.25, -129.75)
  line L350 (-2.25, -129.75) -> (-2.25, -150.25)
  arc A232 (-2.25, -150.25) -> (2.25, -150.25) centre (0, -150.25) ccw
  arc A233 (2.25, -129.75) -> (-2.25, -129.75) centre (0, -129.75) ccw
  line L351 (0, -115.25) -> (0, -94.75) construction
  line L352 (2.25, -115.25) -> (2.25, -94.75)
  line L353 (-2.25, -94.75) -> (-2.25, -115.25)
  arc A234 (-2.25, -115.25) -> (2.25, -115.25) centre (0, -115.25) ccw
  arc A235 (2.25, -94.75) -> (-2.25, -94.75) centre (0, -94.75) ccw
  line L354 (0, -80.25) -> (0, -59.75) construction
  line L355 (2.25, -80.25) -> (2.25, -59.75)
  line L356 (-2.25, -59.75) -> (-2.25, -80.25)
  arc A236 (-2.25, -80.25) -> (2.25, -80.25) centre (0, -80.25) ccw
  arc A237 (2.25, -59.75) -> (-2.25, -59.75) centre (0, -59.75) ccw
  line L357 (0, -45.25) -> (0, -24.75) construction
  line L358 (2.25, -45.25) -> (2.25, -24.75)
  line L359 (-2.25, -24.75) -> (-2.25, -45.25)
  arc A238 (-2.25, -45.25) -> (2.25, -45.25) centre (0, -45.25) ccw
  arc A239 (2.25, -24.75) -> (-2.25, -24.75) centre (0, -24.75) ccw
  line L360 (0, -10.25) -> (0, 10.25) construction
  line L361 (2.25, -10.25) -> (2.25, 10.25)
  line L362 (-2.25, 10.25) -> (-2.25, -10.25)
  arc A240 (-2.25, -10.25) -> (2.25, -10.25) centre (0, -10.25) ccw
  arc A241 (2.25, 10.25) -> (-2.25, 10.25) centre (0, 10.25) ccw
  line L363 (0, 24.75) -> (0, 45.25) construction
  line L364 (2.25, 24.75) -> (2.25, 45.25)
  line L365 (-2.25, 45.25) -> (-2.25, 24.75)
  arc A242 (-2.25, 24.75) -> (2.25, 24.75) centre (0, 24.75) ccw
  arc A243 (2.25, 45.25) -> (-2.25, 45.25) centre (0, 45.25) ccw
  line L366 (0, 59.75) -> (0, 80.25) construction
  line L367 (2.25, 59.75) -> (2.25, 80.25)
  line L368 (-2.25, 80.25) -> (-2.25, 59.75)
  arc A244 (-2.25, 59.75) -> (2.25, 59.75) centre (0, 59.75) ccw
  arc A245 (2.25, 80.25) -> (-2.25, 80.25) centre (0, 80.25) ccw
  line L369 (0, 94.75) -> (0, 115.25) construction
  line L370 (2.25, 94.75) -> (2.25, 115.25)
  line L371 (-2.25, 115.25) -> (-2.25, 94.75)
  arc A246 (-2.25, 94.75) -> (2.25, 94.75) centre (0, 94.75) ccw
  arc A247 (2.25, 115.25) -> (-2.25, 115.25) centre (0, 115.25) ccw
  line L372 (0, 129.75) -> (0, 150.25) construction
  line L373 (2.25, 129.75) -> (2.25, 150.25)
  line L374 (-2.25, 150.25) -> (-2.25, 129.75)
  arc A248 (-2.25, 129.75) -> (2.25, 129.75) centre (0, 129.75) ccw
  arc A249 (2.25, 150.25) -> (-2.25, 150.25) centre (0, 150.25) ccw
  line L375 (0, 164.75) -> (0, 185.25) construction
  line L376 (2.25, 164.75) -> (2.25, 185.25)
  line L377 (-2.25, 185.25) -> (-2.25, 164.75)
  arc A250 (-2.25, 164.75) -> (2.25, 164.75) centre (0, 164.75) ccw
  arc A251 (2.25, 185.25) -> (-2.25, 185.25) centre (0, 185.25) ccw
  line L378 (0, -325.25) -> (0, -304.75) construction
  line L379 (2.25, -325.25) -> (2.25, -304.75)
  line L380 (-2.25, -304.75) -> (-2.25, -325.25)
  arc A252 (-2.25, -325.25) -> (2.25, -325.25) centre (0, -325.25) ccw
  arc A253 (2.25, -304.75) -> (-2.25, -304.75) centre (0, -304.75) ccw
  line L381 (0, -290.25) -> (0, -269.75) construction
  line L382 (2.25, -290.25) -> (2.25, -269.75)
  line L383 (-2.25, -269.75) -> (-2.25, -290.25)
  arc A254 (-2.25, -290.25) -> (2.25, -290.25) centre (0, -290.25) ccw
  arc A255 (2.25, -269.75) -> (-2.25, -269.75) centre (0, -269.75) ccw
  line L384 (0, -255.25) -> (0, -234.75) construction
  line L385 (2.25, -255.25) -> (2.25, -234.75)
  line L386 (-2.25, -234.75) -> (-2.25, -255.25)
  arc A256 (-2.25, -255.25) -> (2.25, -255.25) centre (0, -255.25) ccw
  arc A257 (2.25, -234.75) -> (-2.25, -234.75) centre (0, -234.75) ccw
  line L387 (0, -220.25) -> (0, -199.75) construction
  line L388 (2.25, -220.25) -> (2.25, -199.75)
  line L389 (-2.25, -199.75) -> (-2.25, -220.25)
  arc A258 (-2.25, -220.25) -> (2.25, -220.25) centre (0, -220.25) ccw
  arc A259 (2.25, -199.75) -> (-2.25, -199.75) centre (0, -199.75) ccw
  line L390 (0, -185.25) -> (0, -164.75) construction
  line L391 (2.25, -185.25) -> (2.25, -164.75)
  line L392 (-2.25, -164.75) -> (-2.25, -185.25)
  arc A260 (-2.25, -185.25) -> (2.25, -185.25) centre (0, -185.25) ccw
  arc A261 (2.25, -164.75) -> (-2.25, -164.75) centre (0, -164.75) ccw
  line L393 (0, -150.25) -> (0, -129.75) construction
  line L394 (2.25, -150.25) -> (2.25, -129.75)
  line L395 (-2.25, -129.75) -> (-2.25, -150.25)
  arc A262 (-2.25, -150.25) -> (2.25, -150.25) centre (0, -150.25) ccw
  arc A263 (2.25, -129.75) -> (-2.25, -129.75) centre (0, -129.75) ccw
  line L396 (0, -115.25) -> (0, -94.75) construction
  line L397 (2.25, -115.25) -> (2.25, -94.75)
  line L398 (-2.25, -94.75) -> (-2.25, -115.25)
  arc A264 (-2.25, -115.25) -> (2.25, -115.25) centre (0, -115.25) ccw
  arc A265 (2.25, -94.75) -> (-2.25, -94.75) centre (0, -94.75) ccw
  line L399 (0, -80.25) -> (0, -59.75) construction
  line L400 (2.25, -80.25) -> (2.25, -59.75)
  line L401 (-2.25, -59.75) -> (-2.25, -80.25)
  arc A266 (-2.25, -80.25) -> (2.25, -80.25) centre (0, -80.25) ccw
  arc A267 (2.25, -59.75) -> (-2.25, -59.75) centre (0, -59.75) ccw
  line L402 (0, -45.25) -> (0, -24.75) construction
  line L403 (2.25, -45.25) -> (2.25, -24.75)
  line L404 (-2.25, -24.75) -> (-2.25, -45.25)
  arc A268 (-2.25, -45.25) -> (2.25, -45.25) centre (0, -45.25) ccw
  arc A269 (2.25, -24.75) -> (-2.25, -24.75) centre (0, -24.75) ccw
  line L405 (0, -10.25) -> (0, 10.25) construction
  line L406 (2.25, -10.25) -> (2.25, 10.25)
  line L407 (-2.25, 10.25) -> (-2.25, -10.25)
  arc A270 (-2.25, -10.25) -> (2.25, -10.25) centre (0, -10.25) ccw
  arc A271 (2.25, 10.25) -> (-2.25, 10.25) centre (0, 10.25) ccw
  line L408 (0, 24.75) -> (0, 45.25) construction
  line L409 (2.25, 24.75) -> (2.25, 45.25)
  line L410 (-2.25, 45.25) -> (-2.25, 24.75)
  arc A272 (-2.25, 24.75) -> (2.25, 24.75) centre (0, 24.75) ccw
  arc A273 (2.25, 45.25) -> (-2.25, 45.25) centre (0, 45.25) ccw
  line L411 (0, 59.75) -> (0, 80.25) construction
  line L412 (2.25, 59.75) -> (2.25, 80.25)
  line L413 (-2.25, 80.25) -> (-2.25, 59.75)
  arc A274 (-2.25, 59.75) -> (2.25, 59.75) centre (0, 59.75) ccw
  arc A275 (2.25, 80.25) -> (-2.25, 80.25) centre (0, 80.25) ccw
  line L414 (0, 94.75) -> (0, 115.25) construction
  line L415 (2.25, 94.75) -> (2.25, 115.25)
  line L416 (-2.25, 115.25) -> (-2.25, 94.75)
  arc A276 (-2.25, 94.75) -> (2.25, 94.75) centre (0, 94.75) ccw
  arc A277 (2.25, 115.25) -> (-2.25, 115.25) centre (0, 115.25) ccw
  line L417 (0, 129.75) -> (0, 150.25) construction
  line L418 (2.25, 129.75) -> (2.25, 150.25)
  line L419 (-2.25, 150.25) -> (-2.25, 129.75)
  arc A278 (-2.25, 129.75) -> (2.25, 129.75) centre (0, 129.75) ccw
  arc A279 (2.25, 150.25) -> (-2.25, 150.25) centre (0, 150.25) ccw
  line L420 (0, -360.25) -> (0, -339.75) construction
  line L421 (2.25, -360.25) -> (2.25, -339.75)
  line L422 (-2.25, -339.75) -> (-2.25, -360.25)
  arc A280 (-2.25, -360.25) -> (2.25, -360.25) centre (0, -360.25) ccw
  arc A281 (2.25, -339.75) -> (-2.25, -339.75) centre (0, -339.75) ccw
  line L423 (0, -325.25) -> (0, -304.75) construction
  line L424 (2.25, -325.25) -> (2.25, -304.75)
  line L425 (-2.25, -304.75) -> (-2.25, -325.25)
  arc A282 (-2.25, -325.25) -> (2.25, -325.25) centre (0, -325.25) ccw
  arc A283 (2.25, -304.75) -> (-2.25, -304.75) centre (0, -304.75) ccw
  line L426 (0, -290.25) -> (0, -269.75) construction
  line L427 (2.25, -290.25) -> (2.25, -269.75)
  line L428 (-2.25, -269.75) -> (-2.25, -290.25)
  arc A284 (-2.25, -290.25) -> (2.25, -290.25) centre (0, -290.25) ccw
  arc A285 (2.25, -269.75) -> (-2.25, -269.75) centre (0, -269.75) ccw
  line L429 (0, -255.25) -> (0, -234.75) construction
  line L430 (2.25, -255.25) -> (2.25, -234.75)
  line L431 (-2.25, -234.75) -> (-2.25, -255.25)
  arc A286 (-2.25, -255.25) -> (2.25, -255.25) centre (0, -255.25) ccw
  arc A287 (2.25, -234.75) -> (-2.25, -234.75) centre (0, -234.75) ccw
  line L432 (0, -220.25) -> (0, -199.75) construction
  line L433 (2.25, -220.25) -> (2.25, -199.75)
  line L434 (-2.25, -199.75) -> (-2.25, -220.25)
  arc A288 (-2.25, -220.25) -> (2.25, -220.25) centre (0, -220.25) ccw
  arc A289 (2.25, -199.75) -> (-2.25, -199.75) centre (0, -199.75) ccw
  line L435 (0, -185.25) -> (0, -164.75) construction
  line L436 (2.25, -185.25) -> (2.25, -164.75)
  line L437 (-2.25, -164.75) -> (-2.25, -185.25)
  arc A290 (-2.25, -185.25) -> (2.25, -185.25) centre (0, -185.25) ccw
  arc A291 (2.25, -164.75) -> (-2.25, -164.75) centre (0, -164.75) ccw
  line L438 (0, -150.25) -> (0, -129.75) construction
  line L439 (2.25, -150.25) -> (2.25, -129.75)
  line L440 (-2.25, -129.75) -> (-2.25, -150.25)
  arc A292 (-2.25, -150.25) -> (2.25, -150.25) centre (0, -150.25) ccw
  arc A293 (2.25, -129.75) -> (-2.25, -129.75) centre (0, -129.75) ccw
  line L441 (0, -115.25) -> (0, -94.75) construction
  line L442 (2.25, -115.25) -> (2.25, -94.75)
  line L443 (-2.25, -94.75) -> (-2.25, -115.25)
  arc A294 (-2.25, -115.25) -> (2.25, -115.25) centre (0, -115.25) ccw
  arc A295 (2.25, -94.75) -> (-2.25, -94.75) centre (0, -94.75) ccw
  line L444 (0, -80.25) -> (0, -59.75) construction
  line L445 (2.25, -80.25) -> (2.25, -59.75)
  line L446 (-2.25, -59.75) -> (-2.25, -80.25)
  arc A296 (-2.25, -80.25) -> (2.25, -80.25) centre (0, -80.25) ccw
  arc A297 (2.25, -59.75) -> (-2.25, -59.75) centre (0, -59.75) ccw
  line L447 (0, -45.25) -> (0, -24.75) construction
  line L448 (2.25, -45.25) -> (2.25, -24.75)
  line L449 (-2.25, -24.75) -> (-2.25, -45.25)
  arc A298 (-2.25, -45.25) -> (2.25, -45.25) centre (0, -45.25) ccw
  arc A299 (2.25, -24.75) -> (-2.25, -24.75) centre (0, -24.75) ccw
  line L450 (0, -10.25) -> (0, 10.25) construction
  line L451 (2.25, -10.25) -> (2.25, 10.25)
  line L452 (-2.25, 10.25) -> (-2.25, -10.25)
  arc A300 (-2.25, -10.25) -> (2.25, -10.25) centre (0, -10.25) ccw
  arc A301 (2.25, 10.25) -> (-2.25, 10.25) centre (0, 10.25) ccw
  line L453 (0, 24.75) -> (0, 45.25) construction
  line L454 (2.25, 24.75) -> (2.25, 45.25)
  line L455 (-2.25, 45.25) -> (-2.25, 24.75)
  arc A302 (-2.25, 24.75) -> (2.25, 24.75) centre (0, 24.75) ccw
  arc A303 (2.25, 45.25) -> (-2.25, 45.25) centre (0, 45.25) ccw
  line L456 (0, 59.75) -> (0, 80.25) construction
  line L457 (2.25, 59.75) -> (2.25, 80.25)
  line L458 (-2.25, 80.25) -> (-2.25, 59.75)
  arc A304 (-2.25, 59.75) -> (2.25, 59.75) centre (0, 59.75) ccw
  arc A305 (2.25, 80.25) -> (-2.25, 80.25) centre (0, 80.25) ccw
  line L459 (0, 94.75) -> (0, 115.25) construction
  line L460 (2.25, 94.75) -> (2.25, 115.25)
  line L461 (-2.25, 115.25) -> (-2.25, 94.75)
  arc A306 (-2.25, 94.75) -> (2.25, 94.75) centre (0, 94.75) ccw
  arc A307 (2.25, 115.25) -> (-2.25, 115.25) centre (0, 115.25) ccw
  line L462 (0, -395.25) -> (0, -374.75) construction
  line L463 (2.25, -395.25) -> (2.25, -374.75)
  line L464 (-2.25, -374.75) -> (-2.25, -395.25)
  arc A308 (-2.25, -395.25) -> (2.25, -395.25) centre (0, -395.25) ccw
  arc A309 (2.25, -374.75) -> (-2.25, -374.75) centre (0, -374.75) ccw
  line L465 (0, -360.25) -> (0, -339.75) construction
  line L466 (2.25, -360.25) -> (2.25, -339.75)
  line L467 (-2.25, -339.75) -> (-2.25, -360.25)
  arc A310 (-2.25, -360.25) -> (2.25, -360.25) centre (0, -360.25) ccw
  arc A311 (2.25, -339.75) -> (-2.25, -339.75) centre (0, -339.75) ccw
  line L468 (0, -325.25) -> (0, -304.75) construction
  line L469 (2.25, -325.25) -> (2.25, -304.75)
  line L470 (-2.25, -304.75) -> (-2.25, -325.25)
  arc A312 (-2.25, -325.25) -> (2.25, -325.25) centre (0, -325.25) ccw
  arc A313 (2.25, -304.75) -> (-2.25, -304.75) centre (0, -304.75) ccw
  line L471 (0, -290.25) -> (0, -269.75) construction
  line L472 (2.25, -290.25) -> (2.25, -269.75)
  line L473 (-2.25, -269.75) -> (-2.25, -290.25)
  arc A314 (-2.25, -290.25) -> (2.25, -290.25) centre (0, -290.25) ccw
  arc A315 (2.25, -269.75) -> (-2.25, -269.75) centre (0, -269.75) ccw
  line L474 (0, -255.25) -> (0, -234.75) construction
  line L475 (2.25, -255.25) -> (2.25, -234.75)
  line L476 (-2.25, -234.75) -> (-2.25, -255.25)
  arc A316 (-2.25, -255.25) -> (2.25, -255.25) centre (0, -255.25) ccw
  arc A317 (2.25, -234.75) -> (-2.25, -234.75) centre (0, -234.75) ccw
  line L477 (0, -220.25) -> (0, -199.75) construction
  line L478 (2.25, -220.25) -> (2.25, -199.75)
  line L479 (-2.25, -199.75) -> (-2.25, -220.25)
  arc A318 (-2.25, -220.25) -> (2.25, -220.25) centre (0, -220.25) ccw
  arc A319 (2.25, -199.75) -> (-2.25, -199.75) centre (0, -199.75) ccw
  line L480 (0, -185.25) -> (0, -164.75) construction
  line L481 (2.25, -185.25) -> (2.25, -164.75)
  line L482 (-2.25, -164.75) -> (-2.25, -185.25)
  arc A320 (-2.25, -185.25) -> (2.25, -185.25) centre (0, -185.25) ccw
  arc A321 (2.25, -164.75) -> (-2.25, -164.75) centre (0, -164.75) ccw
  line L483 (0, -150.25) -> (0, -129.75) construction
  line L484 (2.25, -150.25) -> (2.25, -129.75)
  line L485 (-2.25, -129.75) -> (-2.25, -150.25)
  arc A322 (-2.25, -150.25) -> (2.25, -150.25) centre (0, -150.25) ccw
  arc A323 (2.25, -129.75) -> (-2.25, -129.75) centre (0, -129.75) ccw
  line L486 (0, -115.25) -> (0, -94.75) construction
  line L487 (2.25, -115.25) -> (2.25, -94.75)
  line L488 (-2.25, -94.75) -> (-2.25, -115.25)
  arc A324 (-2.25, -115.25) -> (2.25, -115.25) centre (0, -115.25) ccw
  arc A325 (2.25, -94.75) -> (-2.25, -94.75) centre (0, -94.75) ccw
  line L489 (0, -80.25) -> (0, -59.75) construction
  line L490 (2.25, -80.25) -> (2.25, -59.75)
  line L491 (-2.25, -59.75) -> (-2.25, -80.25)
  arc A326 (-2.25, -80.25) -> (2.25, -80.25) centre (0, -80.25) ccw
  arc A327 (2.25, -59.75) -> (-2.25, -59.75) centre (0, -59.75) ccw
  line L492 (0, -45.25) -> (0, -24.75) construction
  line L493 (2.25, -45.25) -> (2.25, -24.75)
  line L494 (-2.25, -24.75) -> (-2.25, -45.25)
  arc A328 (-2.25, -45.25) -> (2.25, -45.25) centre (0, -45.25) ccw
  arc A329 (2.25, -24.75) -> (-2.25, -24.75) centre (0, -24.75) ccw
  line L495 (0, -10.25) -> (0, 10.25) construction
  line L496 (2.25, -10.25) -> (2.25, 10.25)
  line L497 (-2.25, 10.25) -> (-2.25, -10.25)
  arc A330 (-2.25, -10.25) -> (2.25, -10.25) centre (0, -10.25) ccw
  arc A331 (2.25, 10.25) -> (-2.25, 10.25) centre (0, 10.25) ccw
  line L498 (0, 24.75) -> (0, 45.25) construction
  line L499 (2.25, 24.75) -> (2.25, 45.25)
  line L500 (-2.25, 45.25) -> (-2.25, 24.75)
  arc A332 (-2.25, 24.75) -> (2.25, 24.75) centre (0, 24.75) ccw
  arc A333 (2.25, 45.25) -> (-2.25, 45.25) centre (0, 45.25) ccw
  line L501 (0, 59.75) -> (0, 80.25) construction
  line L502 (2.25, 59.75) -> (2.25, 80.25)
  line L503 (-2.25, 80.25) -> (-2.25, 59.75)
  arc A334 (-2.25, 59.75) -> (2.25, 59.75) centre (0, 59.75) ccw
  arc A335 (2.25, 80.25) -> (-2.25, 80.25) centre (0, 80.25) ccw
  line L504 (0, -430.25) -> (0, -409.75) construction
  line L505 (2.25, -430.25) -> (2.25, -409.75)
  line L506 (-2.25, -409.75) -> (-2.25, -430.25)
  arc A336 (-2.25, -430.25) -> (2.25, -430.25) centre (0, -430.25) ccw
  arc A337 (2.25, -409.75) -> (-2.25, -409.75) centre (0, -409.75) ccw
  line L507 (0, -395.25) -> (0, -374.75) construction
  line L508 (2.25, -395.25) -> (2.25, -374.75)
  line L509 (-2.25, -374.75) -> (-2.25, -395.25)
  arc A338 (-2.25, -395.25) -> (2.25, -395.25) centre (0, -395.25) ccw
  arc A339 (2.25, -374.75) -> (-2.25, -374.75) centre (0, -374.75) ccw
  line L510 (0, -360.25) -> (0, -339.75) construction